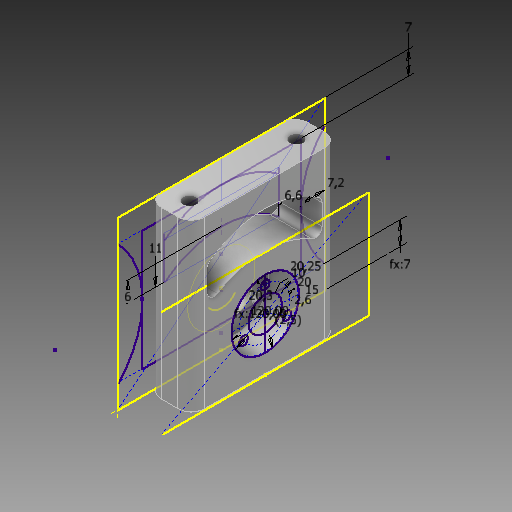
# Autodesk Inventor part: motor_mount_edge
Saved by Autodesk Inventor 2023 (Build 270158000, 158)
## iProperties
Created: 2024-09-10
Part Number: motor_mount_edge
Material: Полиэтилен, низкая плотность
Document SubType Name: Modeling
Designer: Ivan
Density: 0.894 g/cm^3
Appearance: Анодированный — светло-серый
Mass: 15.7548 g
Surface Area: 80.3025 cm^2
Volume: 17.6228 cm^3
Высота: 32,000 мм
Author: Ivan
Autodesk Inventor part; units mm, degrees
ref_plane "YZ Plane" through (0, 0, 0) normal (1, 0, 0) x (0, 1, 0)
ref_plane "XZ Plane" through (0, 0, 0) normal (0, 1, 0) x (-1, 0, 0)
ref_plane "XY Plane" through (0, 0, 0) normal (0, 0, 1) x (1, 0, 0)
sketch "Эскиз1" plane through (0, 0, 0) normal (0, 1, 0) x (-1, 0, 0)
  line L0 (6.5, 31) -> (-6.5, 31)
  line L1 (-6.5, 31) -> (-6.5, -31)
  line L2 (-6.5, -31) -> (6.5, -31)
  line L3 (6.5, -31) -> (6.5, 31)
  line L4 (-6.5, 31) -> (6.5, -31) construction
  line L5 (0, 31) -> (0, -31) construction
  circle A0 centre (0, 16) radius 2
  line L6 (6.5, 0) -> (-6.5, 0) construction
  circle A1 centre (0, -16) radius 2
  point P0 (0, 0)
  point P1 (0, 0)
  dimension "d0" = 13
  dimension "d1" = 62
  dimension "d2" = 16
  dimension "d3" = 4
  constraints: 14 end point, 5 midpoint, 2 centre point, 2 coincident, 2 parallel, 1 horizontal, 1 perpendicular, 1 point on line, 1 symmetric about line, 1 other
  measures "d0" distance of L2.end L1.end
  measures "d1" distance of L0.end L1.end
  measures "d2" distance of point (0, 0) point (0, 16)
  measures "d3" diameter of A0
extrude "Выдавливание1" add sketch "Эскиз1" along normal blind 32
sketch "Эскиз2" plane through (6.5, 0, 31) normal (1, 0, 0) x (0, 0, -1)
  line L0 (0, 32) -> (62, 32)
  line L1 (62, 0) -> (0, 0)
  line L2 (62, 32) -> (0, 0) construction
  circle A0 centre (31, 16) radius 10.15
  line L3 (20.85, 16) -> (41.15, 16) construction
  circle A1 centre (31, 16) radius 10.125
  line L4 (31, 26.125) -> (31, 5.875)
  line L5 (62, 0) -> (62, 32)
  circle A2 centre (31, 16) radius 5
  line L6 (31, 16) -> (24.504809, 12.25) construction
  line L7 (31, 16) -> (37.495191, 12.25) construction
  circle A3 centre (31, 16) radius 7.5 construction
  circle A4 centre (31, 23.5) radius 1.3
  circle A5 centre (37.495191, 12.25) radius 1.3
  circle A6 centre (24.504809, 12.25) radius 1.3
  line L8 (37.495191, 12.25) -> (36.55555, 10.622495) construction
  circle A7 centre (31, 16) radius 10 construction
  line L9 (37.495191, 12.25) -> (39.660254, 11) construction
  point P0 (31, 0)
  dimension "d60" = 20
  dimension "d9" = 20.3
  dimension "d17" = 10
  dimension "d21" = 20.25
  dimension "d57" = 120
  dimension "d58" = 120
  dimension "d59" = 2.6
  dimension "d61" = 2.5
  dimension "d65" = 15
  constraints: 14 end point, 7 centre point, 7 coincident, 7 point on circle, 3 midpoint, 2 equal radius, 1 collinear, 1 horizontal, 1 parallel, 1 perpendicular, 1 point on line, 3 other
  measures "d9" diameter of A0
  measures "d17" diameter of A2
  measures "d21" diameter of A1
  measures "d57" angle of L4 L7
  measures "d58" angle of L6 L4
  measures "d59" diameter of A5
  measures "d61" distance from line of L8 L9.end
  measures "d65" diameter of A3
extrude "Выдавливание3" cut sketch "Эскиз2" against normal through all contours A4 L4 | L4 A4 | A2 L4 | L4 A2 | A5 | A6
sketch "Эскиз2 outline for Выдавливание4" plane through (6.5, 0, 31) normal (1, 0, 0) x (0, 0, -1)
  circle A0 centre (31, 16) radius 10.125
extrude "Выдавливание4" cut sketch "Эскиз2 outline for Выдавливание4" against normal blind 9
sketch "Эскиз3" plane through (0, 32, 0) normal (0, 1, 0) x (1, 0, 0)
  circle A0 centre (0, -16) radius 2 projected
  circle A1 centre (0, 16) radius 2 projected
  point P0 (0, 0)
extrude "Выдавливание5" add sketch "Эскиз3" against normal blind 25
fillet "Сопряжение1" radius 6 2 edges at (6.5, 16, 31) (6.5, 16, -31)
chamfer "Фаска1" distance 1.3 angle 45 3 edges at (-6.5, 12.25, 7.7952) (-6.5, 12.25, -5.1952) (-6.5, 23.5, 1.3)
sketch "Эскиз6" plane through (0, 32, 0) normal (0, 1, 0) x (1, 0, 0)
  arc A0 (6.5, 25) -> (0.5, 31) centre (0.5, 25) ccw projected
  line L0 (0.5, 31) -> (-6.5, 31) projected
  line L1 (-6.5, 31) -> (-6.5, -31) projected
  line L2 (-6.5, -31) -> (0.5, -31) projected
  arc A1 (0.5, -31) -> (6.5, -25) centre (0.5, -25) ccw projected
  line L3 (6.5, -25) -> (6.5, 25) projected
  point P0 (0, 0)
extrude "Выдавливание6" add sketch "Эскиз6" along normal blind 18
sketch "Эскиз7" plane through (0, 50, 0) normal (0, 1, 0) x (1, 0, 0)
  circle A0 centre (0, -16) radius 2 projected
  circle A1 centre (0, 16) radius 2 projected
  point P0 (0, 0)
extrude "Выдавливание7" cut sketch "Эскиз7" against normal blind 7
sketch "Эскиз9" plane through (-6.5, 0, -31) normal (-1, 0, 0) x (0, 0, 1)
  line L0 (0, 0) -> (0, 50)
  line L1 (0, 50) -> (62, 0) construction
  line L2 (7.2, 43) -> (54.8, 43)
  line L3 (54.8, 43) -> (54.8, 7)
  line L4 (54.8, 7) -> (7.2, 7)
  line L5 (7.2, 7) -> (7.2, 43)
  line L6 (0, 50) -> (62, 50)
  line L7 (0, 0) -> (62, 0)
  line L8 (62, 0) -> (62, 50)
  line L9 (62, 0) -> (56, 0)
  line L10 (7.2, 43) -> (0, 43) construction
  line L11 (7.2, 7) -> (0, 7) construction
  line L12 (54.8, 7) -> (62, 7) construction
  line L13 (54.8, 43) -> (62, 43) construction
  arc A0 (0, 7) -> (0, 43) centre (-18.9, 25) ccw
  arc A1 (62, 43) -> (62, 7) centre (80.9, 25) ccw
  line L14 (13.8, 38.870968) -> (48.2, 38.870968) construction
  line L15 (48.2, 38.870968) -> (48.2, 26.15)
  line L16 (48.2, 26.15) -> (13.8, 26.15) construction
  line L17 (13.8, 26.15) -> (13.8, 38.870968)
  line L18 (31, 38.870968) -> (31, 50) construction
  arc A2 (48.2, 26.15) -> (13.8, 26.15) centre (31, 4.496667) ccw
  arc A3 (26.990369, 13.012884) -> (35.009631, 13.012884) centre (31, 16) ccw
  arc A4 (48.2, 37.15) -> (13.8, 37.15) centre (31, 15.496667) ccw
  line L19 (13.8, 37.15) -> (48.2, 37.15) construction
  circle A5 centre (31, 16) radius 10.15 construction
  point P0 (31, 0)
  point P1 (31, 25)
  point P2 (54.8, 25)
  point P3 (7.2, 25)
  point P4 (31, 32.15)
  dimension "d30" = 7
  dimension "d31" = 7
  dimension "d33" = 7.2
  dimension "d42" = 6.6
  dimension "d44" = 11
  dimension "d45" = 6
  constraints: 30 end point, 11 point on circle, 8 point on line, 6 parallel, 5 midpoint, 5 perpendicular, 4 centre point, 2 collinear, 2 horizontal, 1 equal radius, 1 tangent
  measures "d30" distance from line of L2.start L6
  measures "d31" distance from line of L4.end L7
  measures "d33" distance from line of point (7.2, 25) L0
  measures "d42" distance from line of L16.end L5
  measures "d44" distance of L19.end L15.end
  measures "d45" distance from line of point (31, 32.15) L16
extrude "Выдавливание8" cut sketch "Эскиз9" against normal up to surface (13 mm away) contours L0 A0 | A1 L8
extrude "Выдавливание9" cut sketch "Эскиз9" against normal up to surface (13 mm away) contours A4 L2 | L2 A4 L15 A2 L17
fillet "Сопряжение2" radius 2 4 edges at (0, 26.15, 17.2) (0, 26.15, -17.2) (0, 37.15, 17.2) (0, 37.15, -17.2)
sketch "Эскиз11" plane through (0, 50, 0) normal (0, 1, 0) x (1, 0, 0)
  arc A0 (1, -22) -> (-3, -26) centre (1, -26) ccw
  line L0 (-3, -29.486243) -> (-3, -26)
  line L1 (5.457212, -22) -> (-4.601252, -22)
  arc A1 (-3, -29.486243) -> (-1.997801, -32.134486) centre (1, -29.486243) ccw
  arc A2 (-3, -29.486243) -> (-1.997801, -32.134486) centre (1, -29.486243) ccw
  line L2 (-1.997801, -32.134486) -> (17.505015, -54.211602)
  line L3 (6.5, -25) -> (6.5, 25)
  line L4 (5.457212, -22) -> (6.5, -22)
  arc A3 (0.5, -31) -> (6.5, -25) centre (0.5, -25) ccw
  line L5 (-6.5, -31) -> (0.5, -31)
  line L6 (6.5, -31) -> (6.5, 31)
  point P0 (0, 0)
  point P1 (-2.702505, -31)
  point P2 (-2.877907, -22)
  point P3 (0.96893, -22.000121)
  constraints: 2 end point, 1 horizontal, 1 point on line
extrude "Выдавливание10" cut sketch "Эскиз11" against normal up to surface (50 mm away)
mirror "Зеркальное отражение1" about plane through (0, 0, 0) normal (0, 0, 1) of "Выдавливание10"
fillet "Сопряжение3" radius 4 2 edges at (6.5, 25, 22) (6.5, 25, -22)
sketch "Эскиз12" plane through (0, 50, 0) normal (0, 1, 0) x (1, 0, 0)
  circle A0 centre (0, 16) radius 2
  circle A1 centre (0, -16) radius 2
  circle A2 centre (0, -16) radius 2
  line L0 (0, 16) -> (0, -16)
  arc A3 (6.5, 18) -> (2.5, 22) centre (2.5, 18) ccw
  line L1 (6.5, -18) -> (6.5, 18)
  arc A4 (2.5, -22) -> (6.5, -18) centre (2.5, -18) ccw
  arc A5 (-2.5, 22) -> (-6.5, 18) centre (-2.5, 18) ccw
  line L2 (-6.5, -18) -> (-6.5, 18)
  arc A6 (-6.5, -18) -> (-2.5, -22) centre (-2.5, -18) ccw
  arc A7 (6.5, 18) -> (2.5, 22) centre (2.5, 18) ccw
  line L3 (2.5, 22) -> (1, 22)
  arc A8 (-3, 26) -> (1, 22) centre (1, 26) ccw
  line L4 (-3, 26) -> (-3, 29.486243)
  arc A9 (-2.702505, 31) -> (-3, 29.486243) centre (1, 29.486243) ccw
  line L5 (-2.702505, 31) -> (-6.5, 31)
  line L6 (-6.5, 31) -> (-6.5, -31)
  line L7 (-6.5, -31) -> (-2.702505, -31)
  arc A10 (-3, -29.486243) -> (-2.702505, -31) centre (1, -29.486243) ccw
  line L8 (-3, -29.486243) -> (-3, -26)
  arc A11 (1, -22) -> (-3, -26) centre (1, -26) ccw
  line L9 (1, -22) -> (2.5, -22)
  arc A12 (2.5, -22) -> (6.5, -18) centre (2.5, -18) ccw
  line L10 (6.5, -18) -> (6.5, 18)
  circle A13 centre (0, 16) radius 2
  circle A14 centre (0, -16) radius 2
  line L11 (1, 22) -> (2.5, 22)
  line L12 (-2.5, 22) -> (2.5, 22)
  line L13 (2.5, -22) -> (1, -22)
  line L14 (-2.5, -22) -> (1, -22)
  point P0 (0, 0)
  point P1 (1, 22)
  constraints: 8 end point, 6 symmetric about line, 4 point on circle, 2 centre point, 1 collinear, 1 horizontal, 1 vertical, 2 other
extrude "Выдавливание11" cut sketch "Эскиз12" against normal up to surface (50 mm away) contours L12 A5 L6 L5 A9 L4 A8 | A11 L8 A10 L7 L6 A6 L14
chamfer "Фаска2" distance 0.25 angle 45 8 edges at (6.5, 0, 0) (5.3284, 0, -20.8284) (0, 0, -22) (-5.3284, 0, -20.8284) (-6.5, 0, 0) (-5.3284, 0, 20.8284) (0, 0, 22) (5.3284, 0, 20.8284)
chamfer "Фаска3" distance 0.25 angle 45 8 edges at (-6.5, 43.15, 0) (-6.5, 37.0647, 16.9847) (-6.5, 33.06, 17.2) (-6.5, 28.2187, 16.1873) (-6.5, 32.15, 0) (-6.5, 28.2187, -16.1873) (-6.5, 33.06, -17.2) (-6.5, 37.0647, -16.9847)
equation "\"d58\" = d57"
equation "\"d31\" = d30"
